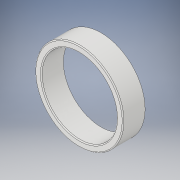
# Autodesk Inventor part: douille
Saved by Autodesk Inventor 2019 (Build 230136000, 136)
## iProperties
Created: 2018-04-25
Part Number: douille
Material: Plastique ABS
Document SubType Name: Modeling
Designer: Theo
Density: 1.06 g/cm^3
Appearance: Lisse - Blanc
Author: Theo
Autodesk Inventor part; units mm, degrees
ref_plane "YZ Plane" through (0, 0, 0) normal (1, 0, 0) x (0, 1, 0)
ref_plane "XZ Plane" through (0, 0, 0) normal (0, 1, 0) x (-1, 0, 0)
ref_plane "XY Plane" through (0, 0, 0) normal (0, 0, 1) x (1, 0, 0)
sketch "Esquisse1" plane through (0, 0, 0) normal (1, 0, 0) x (0, 1, 0)
  line L0 (11.75, 0) -> (10.5, 0)
  line L1 (10.25, -0.25) -> (10.25, -6)
  line L2 (12, -6) -> (12, -0.25)
  line L3 (10, -0.25) -> (10, -17.5) construction
  line L4 (0, 2.9401) -> (0, -22.474)
  line L5 (10.25, -6) -> (12, -6)
  arc A0 (10.5, 0) -> (10.25, -0.25) centre (10.5, -0.25) ccw
  arc A1 (12, -0.25) -> (11.75, 0) centre (11.75, -0.25) ccw
  point P0 (0, 0)
  dimension "d4" = 20
  dimension "d5" = 0.25
  dimension "d6" = 24
  dimension "d30" = 6
  dimension "d63" = 0.25
  dimension "d64" = 0.25
  constraints: 12 end point, 4 point on circle, 4 tangent, 2 centre point, 2 horizontal, 2 horizontal alignment, 2 vertical, 1 parallel, 1 perpendicular, 1 point on line
  measures "d4" diameter of L3 L4
  measures "d5" distance between parallel lines of L1 L3
  measures "d6" diameter of L2 L4
  measures "d30" distance between parallel lines of L5 L0
  measures "d63" radius of A0
  measures "d64" radius of A1
revolve "Révolution1" add sketch "Esquisse1" angle 360 about axis through (0, 0, 2.9401) along (0, 0, -1)
equation "\"d64\" = d63"
